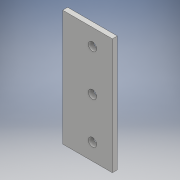
# Autodesk Inventor part: testing_chunk
Saved by Autodesk Inventor 2017.2 (Build 212233000, 233)
## iProperties
Created: 2017-07-25
Part Number: testing_chunk
Material: Generic
Document SubType Name: Modeling
Designer: Nic
Density: 1 g/cm^3
Appearance: Default
Author: Nic
Autodesk Inventor part; units mm, degrees
ref_plane "YZ Plane" through (0, 0, 0) normal (1, 0, 0) x (0, 1, 0)
ref_plane "XZ Plane" through (0, 0, 0) normal (0, 1, 0) x (-1, 0, 0)
ref_plane "XY Plane" through (0, 0, 0) normal (0, 0, 1) x (1, 0, 0)
sketch "Sketch1" plane through (0, 0, 0) normal (0, 1, 0) x (-1, 0, 0)
  line L0 (18, 35) -> (-12, 35)
  line L1 (-12, 35) -> (-12, -35)
  line L2 (-12, -35) -> (18, -35)
  line L3 (18, -35) -> (18, 35)
  circle A0 centre (0, 0) radius 2.5
  circle A1 centre (0, -25) radius 2.5
  circle A2 centre (0, 25) radius 2.5
  dimension "d0" = 5
  dimension "d1" = 25
  dimension "d2" = 25
  dimension "d3" = 10
  dimension "d4" = 10
  dimension "d5" = 30
  dimension "d6" = 12
  constraints: 8 end point, 3 centre point, 2 equal radius, 2 parallel, 2 vertical alignment, 1 coincident, 1 horizontal, 1 perpendicular
  measures "d0" diameter of A0
  measures "d1" distance of A1.centre point (0, 0)
  measures "d2" distance of A2.centre point (0, 0)
  measures "d3" distance from line of L0 A2.centre
  measures "d4" distance from line of L2 A1.centre
  measures "d5" distance between parallel lines of L3 L1
  measures "d6" distance from line of point (0, 0) L1
extrude "Extrusion1" add sketch "Sketch1" along normal blind 3
body "Solid1"
